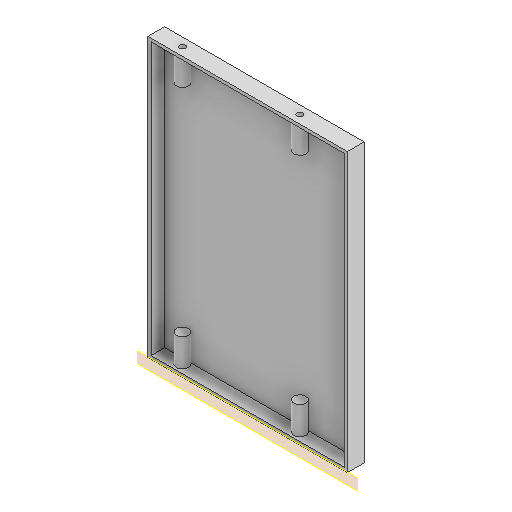
# Autodesk Inventor part: NematostellaImager_illuminationplate
Saved by Autodesk Inventor 2022.5 (Build 265521000, 521)
## iProperties
Created: 2023-11-07
Part Number: NematostellaImager_illuminationplate
Material: Generisch
Document SubType Name: Modeling
Designer: diederichbenedict
Density: 1 g/cm^3
Appearance: Vorgabe
Author: diederichbenedict
Autodesk Inventor part; units mm, degrees
ref_plane "YZ Plane" through (0, 0, 0) normal (1, 0, 0) x (0, 1, 0)
ref_plane "XZ Plane" through (0, 0, 0) normal (0, 1, 0) x (-1, 0, 0)
ref_plane "Arbeitsebene1" through (0, -137.89, 0) normal (0, 0, 1) x (1, 0, 0)
sketch "Skizze1" plane through (0, -137.89, 0) normal (0, 0, 1) x (1, 0, 0)
  line L0 (0, 0) -> (95.3553, 0) projected
  line L1 (95.3553, 0) -> (95.3553, 5) projected
  line L2 (0, 5) -> (95.3553, 5) projected
  line L3 (0, 0) -> (0, 5) projected
  line L4 (0, 137.89) -> (95.3553, 137.89) projected
  line L5 (95.3553, 137.89) -> (95.3553, 142.89) projected
  line L6 (0, 142.89) -> (95.3553, 142.89) projected
  line L7 (0, 137.89) -> (0, 142.89) projected
  line L8 (95.3553, 5) -> (0, 5)
  line L9 (0, 5) -> (0, 137.89)
  line L10 (0, 137.89) -> (95.3553, 137.89)
  line L11 (95.3553, 137.89) -> (95.3553, 5)
  constraints: 8 end point, 2 parallel, 1 horizontal, 1 perpendicular
ref_plane "Arbeitsebene2" through (0, 0, -8) normal (0, 0, -1) x (0, 1, 0)
extrude "Extrusion1" add sketch "Skizze1" against normal up to surface (8 mm away) contours L9 L4 L11 L2
sketch "Skizze2" plane through (0, 0, 0) normal (0, 1, 0) x (1, 0, 0)
  circle A0 centre (68.6881, 4) radius 1.4 projected
  circle A1 centre (12.5176, 4) radius 1.4 projected
  line L0 (0, 0) -> (95.3553, 0) projected
  line L1 (95.3553, 0) -> (95.3553, 68) projected
  line L2 (95.3553, 68) -> (42.0208, 121.3345) projected
  line L3 (42.0208, 121.3345) -> (36.364, 115.6777) projected
  line L4 (36.364, 115.6777) -> (87.3553, 64.6863) projected
  line L5 (87.3553, 64.6863) -> (87.3553, 8) projected
  line L6 (87.3553, 8) -> (0, 8) projected
  line L7 (0, 8) -> (0, 0) projected
  circle A2 centre (42.0208, 115.6777) radius 1.49 projected
  circle A3 centre (72.0208, 85.6777) radius 1.4 projected
  circle A4 centre (57.0208, 100.6777) radius 1.4 projected
hole "Bohrung1" at (68.6881, 0, -4) at (12.5176, 0, -4) direction (0, -1, 0) diameter 2.8 depth 14 tip angle 118
sketch "Skizze3" plane through (0, -132.89, 0) normal (0, -1, 0) x (1, 0, 0)
  circle A0 centre (68.6881, -4) radius 1.4 projected
  circle A1 centre (12.5176, -4) radius 1.4 projected
  line L0 (0, 0) -> (95.3553, 0) projected
  line L1 (0, -8) -> (0, 0) projected
  line L2 (87.3553, -8) -> (0, -8) projected
  line L3 (87.3553, -64.6863) -> (87.3553, -8) projected
  line L4 (36.364, -115.6777) -> (87.3553, -64.6863) projected
  line L5 (42.0208, -121.3345) -> (36.364, -115.6777) projected
  line L6 (95.3553, -68) -> (42.0208, -121.3345) projected
  line L7 (95.3553, 0) -> (95.3553, -68) projected
  circle A2 centre (42.0208, -115.6777) radius 1.49 projected
  circle A3 centre (72.0208, -85.6777) radius 1.4 projected
  circle A4 centre (57.0208, -100.6777) radius 1.4 projected
hole "Bohrung2" at (68.6881, -132.89, -4) at (12.5176, -132.89, -4) direction (0, 1, 0) diameter 2.8 depth 14 tip angle 118
shell "Wandung1" thickness 1.5 removed faces 1 at (63.5702, -44.2967, 0)
